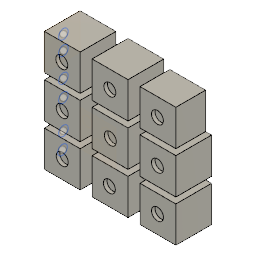
dice v1 (Autodesk Fusion 360 design; units mm, degrees)
Autodesk Fusion 360 part; units mm, degrees
sketch "Sketch1" plane through (0, 0, 0) normal (1, 0, 0) x (0, 0, -1)
sketch "Sketch2" plane through (0, 0, 0) normal (0, 0, 1) x (1, 0, 0)
  line L0 (20, 50) -> (35, 50)
  line L1 (35, 50) -> (35, 35)
  line L2 (35, 35) -> (20, 35)
  line L3 (20, 35) -> (20, 50)
  line L4 (55, 50) -> (55, 35)
  line L5 (55, 35) -> (40, 35)
  line L6 (40, 50) -> (55, 50)
  line L7 (40, 35) -> (40, 50)
  line L8 (75, 50) -> (75, 35)
  line L9 (75, 35) -> (60, 35)
  line L10 (60, 50) -> (75, 50)
  line L11 (60, 35) -> (60, 50)
  line L12 (35, 67.5) -> (35, 52.5)
  line L13 (35, 52.5) -> (20, 52.5)
  line L14 (20, 67.5) -> (35, 67.5)
  line L15 (20, 52.5) -> (20, 67.5)
  line L16 (55, 67.5) -> (55, 52.5)
  line L17 (55, 52.5) -> (40, 52.5)
  line L18 (40, 67.5) -> (55, 67.5)
  line L19 (40, 52.5) -> (40, 67.5)
  line L20 (75, 67.5) -> (75, 52.5)
  line L21 (75, 52.5) -> (60, 52.5)
  line L22 (60, 67.5) -> (75, 67.5)
  line L23 (60, 52.5) -> (60, 67.5)
  line L24 (35, 85) -> (35, 70)
  line L25 (35, 70) -> (20, 70)
  line L26 (20, 85) -> (35, 85)
  line L27 (20, 70) -> (20, 85)
  line L28 (55, 85) -> (55, 70)
  line L29 (55, 70) -> (40, 70)
  line L30 (40, 85) -> (55, 85)
  line L31 (40, 70) -> (40, 85)
  line L32 (75, 85) -> (75, 70)
  line L33 (75, 70) -> (60, 70)
  line L34 (60, 85) -> (75, 85)
  line L35 (60, 70) -> (60, 85)
  dimension "d3" = 40
  dimension "d4" = 35
extrude "Extrude1" add sketch "Sketch2" along normal blind 15 makes body 1 at (25, 50, 5) makes body 2 at (75, 80, 5) makes body 3 at (55, 80, 5) makes body 4 at (35, 62.5, 5) makes body 5 at (55, 45, 5) makes body 6 at (75, 62.5, 5) makes body 7 at (35, 80, 5) makes body 8 at (55, 62.5, 5) makes body 9 at (75, 45, 5)
sketch "Sketch3" plane through (0, 0, 15) normal (0, 0, 1) x (1, 0, 0)
  line L0 (40, 52.5) -> (55, 52.5)
  line L1 (55, 52.5) -> (55, 67.5)
  line L2 (55, 67.5) -> (40, 67.5)
  line L3 (40, 67.5) -> (40, 52.5)
  circle A0 centre (47.6203, 60) radius 2.5
  dimension "d7" = 5
  measures "d7" diameter of A0
sketch "Sketch4" plane through (0, 0, 15) normal (0, 0, 1) x (1, 0, 0)
  line L0 (40, 70) -> (55, 70)
  line L1 (55, 70) -> (55, 85)
  line L2 (55, 85) -> (40, 85)
  line L3 (40, 85) -> (40, 70)
  circle A0 centre (47.4154, 77.6174) radius 2.5
  circle A1 centre (27.3277, 77.5) radius 2.5
  circle A2 centre (67.3062, 77.5) radius 2.5
  circle A3 centre (27.5, 59.8929) radius 2.5023
  circle A4 centre (67.3062, 60) radius 2.5
  circle A5 centre (27.5, 42.5) radius 2.5
  circle A6 centre (47.2185, 42.5) radius 2.5
  circle A7 centre (67.3062, 42.5) radius 2.5
  dimension "d8" = 5
  dimension "d9" = 5
  dimension "d10" = 5
  dimension "d11" = 5
  dimension "d12" = 5
  dimension "d13" = 5
  dimension "d14" = 5
  measures "d8" diameter of A0
  measures "d9" diameter of A1
  measures "d10" diameter of A2
  measures "d11" diameter of A4
  measures "d12" diameter of A5
  measures "d13" diameter of A6
  measures "d14" diameter of A7
extrude "Extrude2" cut sketch "Sketch3" sketch "Sketch4" against normal blind 1.5 contours A0 of sketch 2 contours A0 | A1 | A2 | A3 | A4 | A5 | A6 | A7 bodies 1 2 3 4 5 6 7 8 9
sketch "Sketch5" plane through (0, 0, 0) normal (0, 0, -1) x (-1, 0, 0)
  line L0 (-75, 70) -> (-60, 70)
  line L1 (-60, 70) -> (-60, 85)
  line L2 (-60, 85) -> (-75, 85)
  line L3 (-75, 85) -> (-75, 70)
  circle A0 centre (-72, 81) radius 2
  circle A1 centre (-62.8715, 80.7996) radius 2
  circle A2 centre (-67.3546, 75.0005) radius 2
  circle A3 centre (-51, 81) radius 2
  circle A4 centre (-43, 81) radius 2
  circle A5 centre (-47.4635, 75.1178) radius 2
  circle A6 centre (-31, 80) radius 2.3782
  circle A7 centre (-24, 80) radius 2
  circle A8 centre (-27.4655, 75.0038) radius 2
  circle A9 centre (-71.3128, 63.6217) radius 2
  circle A10 centre (-63, 63) radius 2
  circle A11 centre (-67.6017, 57.5175) radius 2
  circle A12 centre (-51, 64) radius 2
  circle A13 centre (-43, 64) radius 2
  circle A14 centre (-47.3125, 57.519) radius 2
  circle A15 centre (-31.474, 63.9037) radius 2
  circle A16 centre (-23, 64) radius 2
  circle A17 centre (-27.4655, 57.3909) radius 2
  circle A18 centre (-70.8911, 46.1339) radius 2
  circle A19 centre (-63, 46) radius 2
  circle A20 centre (-67.183, 40.003) radius 2
  circle A21 centre (-51, 46) radius 2
  circle A22 centre (-43, 46) radius 2
  circle A23 centre (-47.4236, 40.0084) radius 2
  circle A24 centre (-31, 46) radius 2
  circle A25 centre (-22.9876, 46.3573) radius 2
  circle A26 centre (-27.2911, 40.0087) radius 2
  dimension "d17" = 4
  dimension "d18" = 4
  dimension "d19" = 4
  dimension "d20" = 4
  dimension "d21" = 4
  dimension "d22" = 4
  dimension "d23" = 4
  dimension "d24" = 4
  dimension "d25" = 4
  dimension "d26" = 4
  dimension "d27" = 4
  dimension "d28" = 4
  dimension "d29" = 4
  dimension "d30" = 4
  dimension "d31" = 4
  dimension "d32" = 4
  dimension "d33" = 4
  dimension "d34" = 4
  dimension "d35" = 4
  dimension "d36" = 4
  dimension "d37" = 4
  dimension "d38" = 4
  dimension "d39" = 4
  measures "d17" diameter of A0
  measures "d18" diameter of A1
  measures "d19" diameter of A2
  measures "d20" diameter of A3
  measures "d21" diameter of A5
  measures "d22" diameter of A7
  measures "d23" diameter of A8
  measures "d24" diameter of A9
  measures "d25" diameter of A10
  measures "d26" diameter of A11
  measures "d27" diameter of A12
  measures "d28" diameter of A14
  measures "d29" diameter of A15
  measures "d30" diameter of A16
  measures "d31" diameter of A17
  measures "d32" diameter of A18
  measures "d33" diameter of A20
  measures "d34" diameter of A21
  measures "d35" diameter of A22
  measures "d36" diameter of A23
  measures "d37" diameter of A24
  measures "d38" diameter of A25
  measures "d39" diameter of A26
extrude "Extrude3" cut sketch "Sketch5" against normal blind 2.5 contours L0 L1 L2 L3 | A0 | A1 | A2 | A3 | A4 | A5 | A6 | A7 | A8 | A9 | A10 | A11 | A12 | A13 | A14 | A15 | A16 | A17 | A18 | A19 | A20 | A21 | A22 | A23 | A24 | A25 | A26 bodies 1 2 3 4 5 6 7 8 9
sketch "Sketch6" plane through (0, 0, 2.5) normal (0, 0, -1) x (-1, 0, 0)
  line L0 (-75, 85) -> (-75, 70)
  line L1 (-75, 70) -> (-60, 70)
  line L2 (-60, 70) -> (-60, 85)
  line L3 (-60, 85) -> (-75, 85)
  circle A0 centre (-71, 81) radius 2
  circle A1 centre (-65, 81) radius 2
  circle A2 centre (-68, 74) radius 2
  dimension "d42" = 4
  dimension "d43" = 4
  measures "d42" diameter of A0
  measures "d43" diameter of A2
extrude "Extrude4" cut sketch "Sketch6" against normal blind 2.5 contours A0 | A1 | A2 bodies 2
sketch "Sketch7" plane through (0, 0, 0) normal (0, 0, -1) x (-1, 0, 0)
  circle A0 centre (-31, 46) radius 2
  circle A1 centre (-27.2911, 40.0087) radius 2
  circle A2 centre (-22.9876, 46.3573) radius 2
  line L0 (-35, 35) -> (-20, 35)
  line L1 (-20, 35) -> (-20, 50)
  line L2 (-20, 50) -> (-35, 50)
  line L3 (-35, 50) -> (-35, 35)
sketch "Sketch8" plane through (20, 0, 0) normal (-1, 0, 0) x (0, 0, 1)
  line L0 (0, 85) -> (0, 70)
  line L1 (0, 70) -> (15, 70)
  line L2 (15, 70) -> (15, 85)
  line L3 (15, 85) -> (0, 85)
  circle A0 centre (7, 80) radius 2
  circle A1 centre (7, 74) radius 2
  circle A2 centre (7, 64) radius 2
  circle A3 centre (7, 57) radius 2
  circle A4 centre (7, 45) radius 2
  circle A5 centre (7.3697, 38.2974) radius 2
  dimension "d46" = 4
  dimension "d47" = 4
  dimension "d48" = 4
  dimension "d49" = 4
  dimension "d50" = 4
  dimension "d51" = 4
  measures "d46" diameter of A0
  measures "d47" diameter of A1
  measures "d48" diameter of A2
  measures "d49" diameter of A3
  measures "d50" diameter of A4
  measures "d51" diameter of A5
